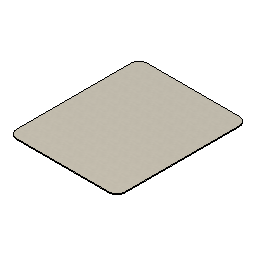
Chassis & Body (Autodesk Fusion 360 archive; units mm, degrees)
design "Bottom plate"
Autodesk Fusion 360 part; units mm, degrees
sketch "Sketch1" plane through (0, 0, 0) normal (0, 1, 0) x (1, 0, 0)
  line L0 (-207.5, 295) -> (207.5, 295)
  line L1 (245, 257.5) -> (245, -257.5)
  line L2 (-245, -257.5) -> (-245, 257.5)
  arc A0 (-207.5, 295) -> (-245, 257.5) centre (-207.5, 257.5) ccw
  arc A1 (245, 257.5) -> (207.5, 295) centre (207.5, 257.5) ccw
  arc A2 (207.5, -295) -> (245, -257.5) centre (207.5, -257.5) ccw
  arc A3 (-245, -257.5) -> (-207.5, -295) centre (-207.5, -257.5) ccw
  line L3 (-207.5, -295) -> (207.5, -295)
  line L4 (-207.5, 257.5) -> (207.5, -257.5) construction
  line L5 (-207.5, -257.5) -> (207.5, 257.5) construction
  point P0 (-245, 295)
  point P1 (245, 295)
  point P2 (-245, -523.5619)
  dimension "d2" = 490
  dimension "d6" = 37.5
  dimension "d10" = 590
  measures "d2" distance of P0 P1
  measures "d6" radius of A0
  measures "d10" distance of L0 L3
extrude "Extrude1" add sketch "Sketch1" along normal blind 4
equation "d2 = 400 mm + 45 mm + 45 mm"
equation "d10 = 500.00 mm + 45 mm + 45 mm"

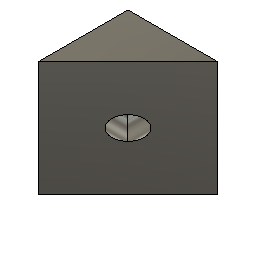
design "45x45 corner piece"
Autodesk Fusion 360 part; units mm, degrees
sketch "Sketch1" plane through (0, 0, 0) normal (0, 1, 0) x (1, 0, 0)
  line L0 (0, 0) -> (35, 0)
  line L1 (35, 0) -> (0, -35)
  line L2 (0, -35) -> (0, 0)
  dimension "d1" = 35
  dimension "d2" = 35
  constraint coincident L0.start L2.end
  constraint horizontal L0
  constraint perpendicular L0 L2
  measures "d1" distance of L0.start L0.end
  measures "d2" distance of L1.end L0.start
extrude "Extrude1" add sketch "Sketch1" along normal blind 45
sketch "Sketch2" plane through (0, 0, 0) normal (-1, 0, 0) x (0, 0, 1)
  line L0 (0, 0) -> (35, 0)
  line L1 (35, 0) -> (35, 45)
  line L2 (35, 45) -> (0, 45)
  line L3 (0, 45) -> (0, 0)
  line L4 (0, 45) -> (35, 0) construction
  circle A0 centre (17.5, 22.5) radius 4.5
  dimension "d5" = 9
  constraint coincident L2.end L3.start
  constraint coincident L0.end L1.start
  constraint midpoint L4 A0.centre
  measures "d5" diameter of A0
extrude "Extrude2" cut sketch "Sketch2" against normal blind 110 contours A0
sketch "Sketch3" plane through (0, 0, 0) normal (0, 0, -1) x (-1, 0, 0)
  line L0 (-35, 0) -> (0, 0)
  line L1 (0, 0) -> (0, 45)
  line L2 (0, 45) -> (-35, 45)
  line L3 (-35, 45) -> (-35, 0)
  line L4 (0, 45) -> (-35, 0) construction
  circle A0 centre (-17.5, 22.5) radius 4.5
  point P0 (0, 22.5)
  dimension "d8" = 9
  constraint coincident L1.end L2.start
  constraint coincident L0.start L3.end
  constraint midpoint L4 A0.centre
  measures "d8" diameter of A0
extrude "Extrude3" cut sketch "Sketch3" against normal blind 45 contours A0
sketch "Sketch4" plane through (0, 0, 0) normal (0, 0, -1) x (-1, 0, 0)
  circle A0 centre (-17.5, 22.5) radius 4.5
  line L0 (-35, 0) -> (0, 0)
  line L1 (0, 0) -> (0, 45)
  line L2 (0, 45) -> (-35, 45)
  line L3 (-35, 45) -> (-35, 0)
  point P0 (0, 22.5)
  constraint coincident L1 P0
  constraint midpoint L1 P0

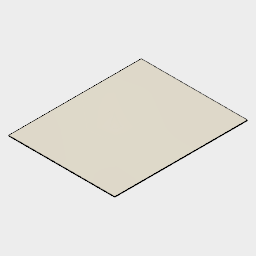
design "Backplate"
Autodesk Fusion 360 part; units mm, degrees
sketch "Sketch1" plane through (0, 0, 0) normal (0, 1, 0) x (1, 0, 0)
  line L0 (0, 0) -> (400, 0)
  line L1 (400, 0) -> (400, -500)
  line L2 (400, -500) -> (0, -500)
  line L3 (0, -500) -> (0, 0)
  dimension "d1" = 400
  dimension "d2" = 500
  constraint horizontal L0
  constraint vertical L1
  constraint horizontal L2
  constraint vertical L3
  constraint coincident L0.start L3.end
extrude "Extrude1" add sketch "Sketch1" along normal blind 2.5

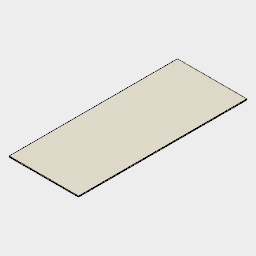
design "Front plate"
Autodesk Fusion 360 part; units mm, degrees
sketch "Sketch1" plane through (0, 0, 0) normal (0, 1, 0) x (1, 0, 0)
  line L0 (0, 0) -> (165, 0)
  line L1 (165, 0) -> (165, -400)
  line L2 (165, -400) -> (0, -400)
  line L3 (0, -400) -> (0, 0)
  dimension "d1" = 165
  dimension "d2" = 400
  constraint horizontal L0
  constraint vertical L1
  constraint horizontal L2
  constraint vertical L3
  constraint coincident L0.start L3.end
extrude "Extrude1" add sketch "Sketch1" along normal blind 2.5

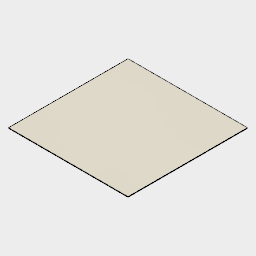
design "Side plate"
Autodesk Fusion 360 part; units mm, degrees
sketch "Sketch1" plane through (0, 0, 0) normal (0, 1, 0) x (1, 0, 0)
  line L0 (0, 0) -> (500, 0)
  line L1 (500, 0) -> (500, -500)
  line L2 (500, -500) -> (0, -500)
  line L3 (0, -500) -> (0, 0)
  dimension "d1" = 500
  dimension "d2" = 500
  constraint horizontal L0
  constraint vertical L1
  constraint horizontal L2
  constraint vertical L3
  constraint coincident L0.start L3.end
extrude "Extrude1" add sketch "Sketch1" along normal blind 2.5

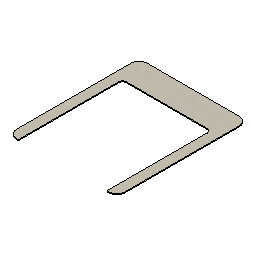
design "Top plate"
Autodesk Fusion 360 part; units mm, degrees
sketch "Sketch1" plane through (0, 0, 0) normal (0, 1, 0) x (1, 0, 0)
  line L0 (37.5, 0) -> (452.5, 0)
  line L1 (490, -37.5) -> (490, -552.7439)
  line L2 (0, -552.5) -> (0, -37.5)
  line L3 (445, -590) -> (445, -137.5)
  line L4 (427.5, -120) -> (62.5, -120)
  line L5 (45, -137.5) -> (45, -590)
  arc A0 (37.5, 0) -> (0, -37.5) centre (37.5, -37.5) ccw
  arc A1 (490, -37.5) -> (452.5, 0) centre (452.5, -37.5) ccw
  arc A2 (451.1619, -590.22) -> (490, -552.7439) centre (452.5, -552.7439) ccw
  arc A3 (0, -552.5) -> (37.5, -590) centre (37.5, -552.5) ccw
  arc A4 (62.5, -120) -> (45, -137.5) centre (62.5, -137.5) ccw
  arc A5 (445, -137.5) -> (427.5, -120) centre (427.5, -137.5) ccw
  line L6 (445, -590) -> (451.1619, -590.22)
  line L7 (37.5, -590) -> (45, -590)
  point P0 (490, 0)
  dimension "d1" = 45
  dimension "width" = 490
  dimension "d4" = 45
  dimension "d5" = 120
  dimension "d6" = 37.5
  dimension "d9" = 17.5
  dimension "length" = 590
  dimension "d11" = 590
  constraint horizontal L0
  constraint vertical L1
  constraint vertical L2
  constraint vertical L3
  constraint horizontal L4
  constraint vertical L5
  constraint coincident origin L0
  constraint coincident origin L2
  constraint tangent L0 A0
  constraint tangent L2 A0
  constraint coincident P0 L0
  constraint coincident P0 L1
  constraint tangent L0 A1
  constraint tangent L1 A1
  constraint equal A0 A1
  constraint tangent L1 A2
  constraint equal A0 A2
  constraint tangent L2 A3
  constraint equal A0 A3
  constraint tangent L4 A4
  constraint tangent L5 A4
  constraint tangent L3 A5
  constraint tangent L4 A5
  constraint equal A4 A5
  constraint coincident L3 L6.start
  constraint tangent A2 L6
  constraint coincident L3.start L6.start
  constraint horizontal L7
  constraint coincident L5.end L7.end
  constraint tangent A3 L7
  measures "d1" distance of L1 L3
  measures "width" distance of origin P0
  measures "d4" distance of L2 L5
  measures "d5" distance of L0 L4
  measures "d6" radius of A0
  measures "d9" radius of A4
  measures "length" distance of L0 L5.end
  measures "d11" distance of L0 L3.start
extrude "Extrude1" add sketch "Sketch1" along normal blind 4
ref_plane "WorkPlane1" through (245, 0, 0) normal (1, 0, 0) x (0, 1, 0)
equation "width = 400 mm + 45 mm + 45 mm"
equation "length = 500.00 mm + 45 mm + 45 mm"
equation "d11 = length"
equation "d12 = width / 2"
equation "d13 = 31 mm"
equation "d14 = d13"
equation "d16 = 5.5 mm"
equation "d17 = d16"
equation "d18 = d16"
equation "d19 = d16"
equation "d21 = ( 45.00 mm - d13 - d18 - d17 ) / 2"
